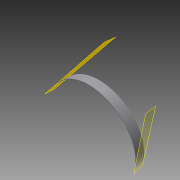
# Autodesk Inventor part: curvedTrack
Saved by Autodesk Inventor 2011 SP1 (Build 150282100, 282)
## iProperties
Created: 2013-01-18
Part Number: curvedTrack
Document SubType Name: Modeling
Designer: wes
Density: 1 g/cm^3
Author: wes
Autodesk Inventor part; units mm, degrees
ref_plane "YZ Plane" through (0, 0, 0) normal (1, 0, 0) x (0, 1, 0)
ref_plane "XZ Plane" through (0, 0, 0) normal (0, 1, 0) x (-1, 0, 0)
ref_plane "XY Plane" through (0, 0, 0) normal (0, 0, 1) x (1, 0, 0)
sketch "Sketch1" plane through (0, 0, 0) normal (0, 0, 1) x (1, 0, 0)
  arc A0 (380.5355, -38.0375) -> (-270.1768, 230.7579) centre (4.8231, -25.5444) ccw
  arc A1 (383.5416, -39.2939) -> (-271.6172, 233.6803) centre (4.8231, -25.5444) ccw
  line L0 (-271.6172, 233.6803) -> (-270.1768, 230.7579)
  line L1 (380.5355, -38.0375) -> (383.5416, -39.2939)
  point P0 (0, 0)
  dimension "d0" = 375.92
  dimension "d1" = 138.92
  dimension "d3" = 138.92
  dimension "d4" = 378.968
  constraints: 4 end point, 4 point on circle, 2 centre point, 1 coincident
  measures "d0" radius of A0
  measures "d4" radius of A1
extrude "Extrusion1" add sketch "Sketch1" along normal blind 76.2
ref_plane "Work Plane3" through (383.5416, -39.2939, 0) normal (0.9993, -0.0363, 0) x (0.0363, 0.9993, 0)
ref_plane "Work Plane4" through (-271.6172, 233.6803, 0) normal (-0.7295, 0.684, 0) x (-0.684, -0.7295, 0)
equation "\"d3\" = d1"
body "Solid1"
